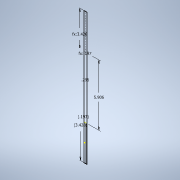
# Autodesk Inventor part: Mount
Saved by Autodesk Inventor 2020 (Build 240168000, 168)
## iProperties
Created: 2020-03-06
Part Number: Mount
Material: Generic
Document SubType Name: Modeling
Designer: Sverrir
Density: 1 g/cm^3
Appearance: Default
Author: Sverrir
Autodesk Inventor part; units mm, degrees
ref_plane "YZ Plane" through (0, 0, 0) normal (1, 0, 0) x (0, 1, 0)
ref_plane "XZ Plane" through (0, 0, 0) normal (0, 1, 0) x (-1, 0, 0)
ref_plane "XY Plane" through (0, 0, 0) normal (0, 0, 1) x (1, 0, 0)
sketch "Sketch1" plane through (0, 0, 0) normal (0, 0, 1) x (1, 0, 0)
  line L0 (2.5, -43.5378) -> (2.5, 43.5378) construction
  line L1 (2.5, 43.5378) -> (-2.5, 43.5378) projected
  line L2 (-2.5, 43.5378) -> (-2.5, -43.5378) projected
  line L3 (-2.5, -43.5378) -> (2.5, -43.5378) projected
  line L4 (-2.5, -43.5378) -> (2.5, -43.5378)
  line L5 (2.5, -43.5378) -> (2.5, 43.5378)
  line L6 (2.5, 43.5378) -> (-2.5, 43.5378) construction
  line L7 (-2.5, 43.5378) -> (-2.5, -43.5378)
  line L8 (-2.5, 193.5378) -> (2.5, 193.5378) construction
  line L9 (2.5, 193.5378) -> (2.5, 280.6134) construction
  line L10 (2.5, 280.6134) -> (-2.5, 280.6134)
  line L11 (-2.5, 280.6134) -> (-2.5, 193.5378)
  line L12 (-2.5, -43.5378) -> (5, -43.5378)
  line L13 (5, -43.5378) -> (5, 280.6134)
  line L14 (5, 280.6134) -> (-2.5, 280.6134)
  line L15 (-2.5, 280.6134) -> (-2.5, -43.5378)
  point P0 (0, 0)
  dimension "d0" = 5
  dimension "d1" = 5
  dimension "d2" = 87.0756
  dimension "d3" = 87.0756
  dimension "d4" = 150
  dimension "d5" = 7.5
  constraints: 24 end point, 6 parallel, 3 horizontal, 3 perpendicular, 1 collinear, 1 point on line
  measures "d0" distance of L8.start L8.end
  measures "d1" distance of L0.end L1.end
  measures "d2" distance of L1.end L2.end
  measures "d3" distance of L10.end L8.start
  measures "d4" distance between parallel lines of L8 L1
  measures "d5" distance between parallel lines of L15 L13
extrude "Extrusion1" add sketch "Sketch1" along normal blind 19.05
equation "\"d0\" = d1"
equation "\"d3\" = d2"
body "Solid1"
